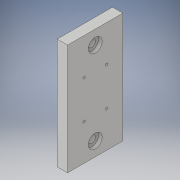
# Autodesk Inventor part: FV mounting plate V1
Saved by Autodesk Inventor 2019 (Build 230136000, 136)
## iProperties
Created: 2019-01-04
Part Number: FV mounting plate V1
Material: Generic
Document SubType Name: Modeling
Designer: dewanlab
Density: 1 g/cm^3
Appearance: Default
Author: dewanlab
Autodesk Inventor part; units mm, degrees
ref_plane "YZ Plane" through (0, 0, 0) normal (1, 0, 0) x (0, 1, 0)
ref_plane "XZ Plane" through (0, 0, 0) normal (0, 1, 0) x (-1, 0, 0)
ref_plane "XY Plane" through (0, 0, 0) normal (0, 0, 1) x (1, 0, 0)
sketch "Sketch1" plane through (0, 0, 0) normal (1, 0, 0) x (0, 1, 0)
  line L0 (74.1326, 23.8494) -> (-27.4674, 23.8494)
  line L1 (-27.4674, 23.8494) -> (-27.4674, -26.9506)
  line L2 (-27.4674, -26.9506) -> (74.1326, -26.9506)
  line L3 (74.1326, -26.9506) -> (74.1326, 23.8494)
  point P0 (0, 0)
  dimension "d0" = 50.8
  dimension "d1" = 101.6
  constraints: 8 end point, 2 parallel, 1 horizontal, 1 perpendicular
  measures "d0" distance between parallel lines of L2 L0
  measures "d1" distance between parallel lines of L1 L3
extrude "Extrusion1" add sketch "Sketch1" along normal blind 9.525
sketch "Sketch2" plane through (9.525, 0, 0) normal (1, 0, 0) x (0, 0, -1)
  line L0 (-23.8494, 74.1326) -> (-23.8494, -27.4674) projected
  line L1 (26.9506, 74.1326) -> (-23.8494, 74.1326) projected
  point P0 (0, 0)
  point P1 (1.5506, 61.4326)
  dimension "d11" = 25.4
  dimension "d12" = 12.7
  measures "d11" distance from line of L0 point (1.551, 61.433)
  measures "d12" distance from line of L1 point (1.551, 61.433)
hole "Hole1" at (9.525, 61.4326, -1.5506) direction (-1, 0, 0) diameter 6.7564 end through all counterbore diameter 12.7 counterbore depth 3.175
sketch "Sketch3" plane through (9.525, 0, 0) normal (1, 0, 0) x (0, 0, -1)
  line L0 (-23.8494, 74.1326) -> (-23.8494, -27.4674) projected
  line L1 (-23.8494, -27.4674) -> (26.9506, -27.4674) projected
  point P0 (0, 0)
  point P1 (1.5506, -14.7674)
  dimension "d21" = 25.4
  dimension "d22" = 12.7
  measures "d21" distance from line of L0 point (1.551, -14.767)
  measures "d22" distance from line of L1 point (1.551, -14.767)
hole "Hole2" at (9.525, -14.7674, -1.5506) direction (-1, 0, 0) diameter 6.7564 end through all counterbore diameter 12.7 counterbore depth 3.175
sketch "Sketch4" plane through (0, 0, 0) normal (-1, 0, 0) x (0, 0, 1)
  line L0 (-26.9506, 74.1326) -> (23.8494, 74.1326) projected
  line L1 (23.8494, 74.1326) -> (23.8494, -27.4674) projected
  point P0 (0, 0)
  point P1 (8.7364, 40.8586)
  dimension "d30" = 33.274
  dimension "d31" = 15.113
  measures "d30" distance from line of point (8.736, 40.859) L0
  measures "d31" distance from line of L1 point (8.736, 40.859)
hole "Hole3" at (0, 40.8586, 8.7364) direction (1, 0, 0) diameter 2.159 end through all counterbore diameter 5.08 counterbore depth 1.651
sketch "Sketch5" plane through (0, 0, 0) normal (-1, 0, 0) x (0, 0, 1)
  line L0 (23.8494, -27.4674) -> (-26.9506, -27.4674) projected
  line L1 (-26.9506, 74.1326) -> (23.8494, 74.1326) projected
  line L2 (23.8494, 74.1326) -> (23.8494, -27.4674) projected
  point P0 (0, 0)
  point P1 (8.7364, 5.8066)
  dimension "d41" = 33.274
  dimension "d42" = 15.113
  measures "d41" distance from line of L0 point (8.736, 5.807)
  measures "d42" distance from line of L2 point (8.736, 5.807)
hole "Hole4" at (0, 5.8066, 8.7364) direction (1, 0, 0) diameter 2.159 end through all counterbore diameter 5.08 counterbore depth 1.651
sketch "Sketch6" plane through (0, 0, 0) normal (-1, 0, 0) x (0, 0, 1)
  line L0 (-26.9506, -27.4674) -> (-26.9506, 74.1326) projected
  line L1 (-26.9506, 74.1326) -> (23.8494, 74.1326) projected
  point P0 (0, 0)
  point P1 (-11.8376, 40.8586)
  dimension "d50" = 15.113
  dimension "d51" = 33.274
  measures "d50" distance from line of L0 point (-11.838, 40.859)
  measures "d51" distance from line of L1 point (-11.838, 40.859)
hole "Hole5" at (0, 40.8586, -11.8376) direction (1, 0, 0) diameter 2.159 end through all counterbore diameter 5.08 counterbore depth 1.651
sketch "Sketch7" plane through (0, 0, 0) normal (-1, 0, 0) x (0, 0, 1)
  line L0 (-26.9506, -27.4674) -> (-26.9506, 74.1326) projected
  line L1 (23.8494, -27.4674) -> (-26.9506, -27.4674) projected
  point P0 (0, 0)
  point P1 (-11.8376, 5.8066)
  dimension "d59" = 15.113
  dimension "d60" = 33.274
  measures "d59" distance from line of L0 point (-11.838, 5.807)
  measures "d60" distance from line of L1 point (-11.838, 5.807)
hole "Hole6" at (0, 5.8066, -11.8376) direction (1, 0, 0) diameter 2.159 end through all counterbore diameter 5.08 counterbore depth 1.651
body "Solid1"
